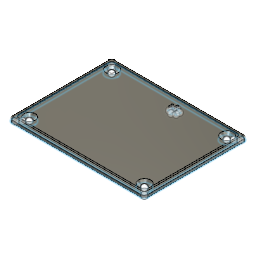
iot-data-logger-enclosure-top-cover v9 (Autodesk Fusion 360 design; units mm, degrees)
Autodesk Fusion 360 part; units mm, degrees
sketch "Sketch1" plane through (0, 0, 0) normal (0, 1, 0) x (1, 0, 0)
  line L0 (2, 0) -> (77, 0)
  line L1 (79, -1.9978) -> (79, -58)
  line L2 (77, -60) -> (2, -60)
  line L3 (0, -58) -> (0, -2)
  arc A0 (2, 0) -> (0, -2) centre (2, -2) ccw
  arc A1 (0, -58) -> (2, -60) centre (2, -58) ccw
  arc A2 (77, -60) -> (79, -58) centre (77, -58) ccw
  arc A3 (79, -2.0022) -> (77, 0) centre (77, -2) ccw
  circle A4 centre (6, -6) radius 1.5
  circle A5 centre (6, -6) radius 3.5
  circle A6 centre (6, -54) radius 3.5
  circle A7 centre (73, -54) radius 3.5
  circle A8 centre (73, -6) radius 3.5
  line L4 (4, -2) -> (75, -2)
  line L5 (77, -4) -> (77, -56)
  line L6 (75, -58) -> (4, -58)
  line L7 (2, -56) -> (2, -4)
  arc A9 (75, -58) -> (77, -56) centre (75, -56) ccw
  arc A10 (2, -56) -> (4, -58) centre (4, -56) ccw
  arc A11 (4, -2) -> (2, -4) centre (4, -4) ccw
  arc A12 (77, -4) -> (75, -2) centre (75, -4) ccw
  circle A13 centre (73, -6) radius 1.5
  circle A14 centre (73, -54) radius 1.5
  circle A15 centre (6, -54) radius 1.5
  line L8 (44, -5) -> (44, -9)
  line L9 (43, -9) -> (43, -5)
  line L10 (46, -6) -> (46, -8)
  line L11 (45, -8) -> (45, -6)
  line L12 (42, -6) -> (42, -8)
  line L13 (41, -8) -> (41, -6)
  arc A16 (42, -6) -> (41, -6) centre (41.5, -6) ccw
  arc A17 (41, -8) -> (42, -8) centre (41.5, -8) ccw
  arc A18 (43, -9) -> (44, -9) centre (43.5, -9) ccw
  arc A19 (44, -5) -> (43, -5) centre (43.5, -5) ccw
  arc A20 (46, -6) -> (45, -6) centre (45.5, -6) ccw
  arc A21 (45, -8) -> (46, -8) centre (45.5, -8) ccw
  dimension "d5" = 67
  dimension "d6" = 48
  dimension "d7" = 3
  dimension "d8" = 7
  dimension "d9" = 7
  dimension "d10" = 3
  constraint horizontal L0
  constraint vertical L1
  constraint horizontal L2
  constraint vertical L3
  constraint tangent L0 A0
  constraint tangent L2 A1
  constraint tangent L1 A2
  constraint tangent L0 A3
  constraint coincident L1.start A3
  constraint coincident L1 A3.start
  constraint horizontal L4
  constraint vertical L5
  constraint horizontal L6
  constraint vertical L7
  constraint tangent L5 A9
  constraint tangent L6 A10
  constraint tangent L4 A11
  constraint tangent L4 A12
  constraint concentric A8 A13
  constraint concentric A7 A14
  constraint concentric A6 A15
  constraint vertical L8
  constraint vertical L9
  constraint vertical L10
  constraint vertical L11
  constraint vertical L12
  constraint vertical L13
  measures "d5" distance of A4.centre A8.centre
  measures "d6" distance of A4.centre A6.centre
  measures "d7" diameter of A4
  measures "d8" diameter of A5
  measures "d9" diameter of A6
  measures "d10" diameter of A14
extrude "Extrude7" add sketch "Sketch1" along normal blind 2.5 contours L0 L1 L2 L3 A0 A1 A2 A3
extrude "Extrude8" add sketch "Sketch1" along normal blind 2 contours A4 | A5 | A6 | A7 | A8 | L4 L5 L6 L7 A9 A10 A11 A12 | A13 | A14 | A15
hole "Hole7" at (6.0885, 2, 53.8207) direction (0, -1, 0) diameter 3 depth 2 tip angle 180 countersink diameter 6.6 countersink angle 90
hole "Hole8" at (73.0594, 2, 53.841) direction (0, -1, 0) diameter 3 depth 2 tip angle 180 countersink diameter 7 countersink angle 90
hole "Hole9" at (72.9927, 2, 5.7576) direction (0, -1, 0) diameter 3 depth 2 tip angle 180 countersink diameter 7 countersink angle 90
hole "Hole10" at (6.0744, 2, 5.8172) direction (0, -1, 0) diameter 3 depth 2 tip angle 180 countersink diameter 7 countersink angle 90
fillet "Fillet2" radius 1 8 edges at (0, 2.5, 30) (0.5858, 2.5, 59.4142) (39.5, 2.5, 60) (78.4142, 2.5, 59.4142) (79, 2.5, 30.0011) (78.415, 2.5, 0.5866) (39.5, 2.5, 0) (0.5858, 2.5, 0.5858)
hole "Hole6" [rolled back] hole depth 2 hole diameter 3 tip angle 180 csdiameter 7 csangle 90
hole "Hole5" [rolled back] hole depth 2 hole diameter 3 tip angle 180 csdiameter 7 csangle 90
extrude "Extrude1" [rolled back] along distance 2.5 taper angle 0
extrude "Extrude2" [rolled back] along distance 2 taper angle 0
fillet "Fillet1" [rolled back] radius 1
extrude "Extrude3" [rolled back] along distance 2 taper angle 0
hole "Hole1" [rolled back] hole depth 2 hole diameter 3 tip angle 180 csdiameter 7 csangle 90
extrude "Extrude4" [rolled back] along distance 2 taper angle 0
extrude "Extrude5" [rolled back] along distance 2 taper angle 0
extrude "Extrude6" [rolled back] along distance 2 taper angle 0
hole "Hole2" [rolled back] hole depth 2 hole diameter 3 tip angle 180 csdiameter 7 csangle 90
hole "Hole3" [rolled back] hole depth 2 hole diameter 3 tip angle 180 csdiameter 7 csangle 90
hole "Hole4" [rolled back] hole depth 2 hole diameter 3 tip angle 180 csdiameter 7 csangle 90
delete_face "DeleteFace1" [rolled back]
